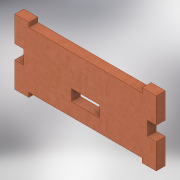
# Autodesk Inventor part: boxBack
Saved by Autodesk Inventor 2017 (Build 210142000, 142)
## iProperties
Created: 2017-05-22
Part Number: boxBack
Material: Generic
Document SubType Name: Modeling
Designer: Dominic Gaiero
Density: 1 g/cm^3
Appearance: Walnut - Natural Polished
Author: Dominic Gaiero
Autodesk Inventor part; units mm, degrees
ref_plane "YZ Plane" through (0, 0, 0) normal (1, 0, 0) x (0, 1, 0)
ref_plane "XZ Plane" through (0, 0, 0) normal (0, 1, 0) x (-1, 0, 0)
ref_plane "XY Plane" through (0, 0, 0) normal (0, 0, 1) x (1, 0, 0)
sketch "Sketch1" plane through (0, 0, 0) normal (0, 0, 1) x (1, 0, 0)
  line L0 (90.8, 43.3229) -> (90.8, 46.4979)
  line L1 (90.8, 46.4979) -> (100.8, 46.4979)
  line L2 (100.8, 46.4979) -> (100.8, 43.175)
  line L3 (94.45, 28.3229) -> (94.45, 18.3229)
  line L4 (90.8, 0.1479) -> (100.8, 0.1479)
  line L5 (100.8, 0.1479) -> (100.8, 6.35)
  line L6 (100.8, 6.35) -> (100.8, 18.3229)
  line L7 (94.45, 18.3229) -> (100.8, 18.3229)
  line L8 (100.8, 28.3229) -> (94.45, 28.3229)
  line L9 (100.8, 28.3229) -> (100.8, 43.175)
  line L10 (90.8, 3.3229) -> (90.8, 0.1479)
  line L11 (10, 3.3229) -> (90.8, 3.3229)
  line L12 (90.8, 43.3229) -> (10, 43.3229)
  line L13 (10, 43.3229) -> (10, 46.4979)
  line L14 (10, 46.4979) -> (0, 46.4979)
  line L15 (0, 46.4979) -> (0, 43.175)
  line L16 (10, 3.3229) -> (10, 0.1479)
  line L17 (6.35, 28.3229) -> (6.35, 18.3229)
  line L18 (0, 43.175) -> (0, 28.3229)
  line L19 (0, 28.3229) -> (6.35, 28.3229)
  line L20 (0, 18.3229) -> (0, 6.35)
  line L21 (6.35, 18.3229) -> (0, 18.3229)
  line L22 (0, 0.1479) -> (0, 6.35)
  line L23 (10, 0.1479) -> (0, 0.1479)
  line L24 (40.4, 20.8229) -> (60.4, 20.8229)
  line L25 (60.4, 20.8229) -> (60.4, 12.8229)
  line L26 (60.4, 12.8229) -> (40.4, 12.8229)
  line L27 (40.4, 12.8229) -> (40.4, 20.8229)
  line L28 (50.4, 43.3229) -> (50.4, 3.3229)
  point P0 (0, 0)
  point P1 (4.5679, 28.3229)
  point P2 (50.4, 12.8229)
  point P3 (6.35, 23.3229)
  point P4 (50.4, 23.3229)
  point P5 (94.45, 23.3229)
  dimension "d0" = 40
  dimension "d1" = 20
  dimension "d2" = 8
  dimension "d3" = 88.1
  dimension "d4" = 80.8
  dimension "d5" = 3.175
  dimension "d6" = 3.175
  dimension "d7" = 3.175
  dimension "d8" = 3.175
  dimension "d9" = 10
  dimension "d10" = 10
  dimension "d11" = 9.5
  constraints: 58 end point, 13 parallel, 6 midpoint, 5 perpendicular, 4 horizontal, 3 horizontal alignment, 1 coincident, 1 vertical, 1 vertical alignment
  measures "d0" distance between parallel lines of L11 L12
  measures "d1" distance of L25.end L26.end
  measures "d2" distance of L25.start L25.end
  measures "d3" distance between parallel lines of L3 L17
  measures "d4" distance between parallel lines of L10 L16
  measures "d5" distance between parallel lines of L12 L14
  measures "d6" distance between parallel lines of L12 L1
  measures "d7" distance between parallel lines of L11 L23
  measures "d8" distance between parallel lines of L11 L4
  measures "d9" distance of L17.start L17.end
  measures "d10" distance of L3.start L3.end
  measures "d11" distance between parallel lines of L11 L26
extrude "Extrusion1" add sketch "Sketch1" along normal blind 6.35
extrude "Extrusion2" cut sketch "Sketch1" along normal blind 6.35 contours L28 L26 L27 L24 | L24 L25 L26 L28
body "Solid1"
